Lower - Final v7 (Autodesk Fusion 360 design; units mm, degrees)
Autodesk Fusion 360 part; units mm, degrees
note: some values were not read from the file. Chosen so that the rebuilt part matches the saved one: which bodies a step acts on; which face or edge a step refers to; the sign of a taper.
sketch "Sketch1" plane through (0, 0, 0) normal (0, 1, 0) x (1, 0, 0)
  line L0 (-39.5, 47.5) -> (39.5, 47.5)
  line L1 (49.5, 37.5) -> (49.5, -37.5)
  line L2 (39.5, -47.5) -> (-39.5, -47.5)
  line L3 (-49.5, -37.5) -> (-49.5, 37.5)
  line L4 (-49.5, 47.5) -> (49.5, -47.5) construction
  line L5 (49.5, 47.5) -> (-49.5, -47.5) construction
  arc A0 (-39.5, 47.5) -> (-49.5, 37.5) centre (-39.5, 37.5) ccw
  arc A1 (49.5, 37.5) -> (39.5, 47.5) centre (39.5, 37.5) ccw
  arc A2 (39.5, -47.5) -> (49.5, -37.5) centre (39.5, -37.5) ccw
  arc A3 (-49.5, -37.5) -> (-39.5, -47.5) centre (-39.5, -37.5) ccw
  line L6 (-46.5, -37.5) -> (-46.5, 37.5)
  arc A4 (-39.5, 44.5) -> (-46.5, 37.5) centre (-39.5, 37.5) ccw
  line L7 (-39.5, 44.5) -> (39.5, 44.5)
  arc A5 (46.5, 37.5) -> (39.5, 44.5) centre (39.5, 37.5) ccw
  line L8 (46.5, 37.5) -> (46.5, -37.5)
  arc A6 (39.5, -44.5) -> (46.5, -37.5) centre (39.5, -37.5) ccw
  line L9 (39.5, -44.5) -> (-39.5, -44.5)
  arc A7 (-46.5, -37.5) -> (-39.5, -44.5) centre (-39.5, -37.5) ccw
  line L10 (-44, -37.5) -> (-44, 37.5)
  arc A8 (-39.5, 42) -> (-44, 37.5) centre (-39.5, 37.5) ccw
  line L11 (-39.5, 42) -> (39.5, 42)
  arc A9 (44, 37.5) -> (39.5, 42) centre (39.5, 37.5) ccw
  line L12 (44, 37.5) -> (44, -37.5)
  arc A10 (39.5, -42) -> (44, -37.5) centre (39.5, -37.5) ccw
  line L13 (39.5, -42) -> (-39.5, -42)
  arc A11 (-44, -37.5) -> (-39.5, -42) centre (-39.5, -37.5) ccw
  line L14 (-47, -37.5) -> (-47, 37.5)
  arc A12 (-39.5, 45) -> (-47, 37.5) centre (-39.5, 37.5) ccw
  line L15 (-39.5, 45) -> (39.5, 45)
  arc A13 (47, 37.5) -> (39.5, 45) centre (39.5, 37.5) ccw
  line L16 (47, 37.5) -> (47, -37.5)
  arc A14 (39.5, -45) -> (47, -37.5) centre (39.5, -37.5) ccw
  line L17 (39.5, -45) -> (-39.5, -45)
  arc A15 (-47, -37.5) -> (-39.5, -45) centre (-39.5, -37.5) ccw
  arc A16 (-39.5, 44.4) -> (-46.4, 37.5) centre (-39.5, 37.5) ccw
  line L18 (-46.4, -37.5) -> (-46.4, 37.5)
  arc A17 (-46.4, -37.5) -> (-39.5, -44.4) centre (-39.5, -37.5) ccw
  line L19 (39.5, -44.4) -> (-39.5, -44.4)
  arc A18 (39.5, -44.4) -> (46.4, -37.5) centre (39.5, -37.5) ccw
  line L20 (46.4, 37.5) -> (46.4, -37.5)
  arc A19 (46.4, 37.5) -> (39.5, 44.4) centre (39.5, 37.5) ccw
  line L21 (-39.5, 44.4) -> (39.5, 44.4)
  arc A20 (-39.5, 44.15) -> (-46.15, 37.5) centre (-39.5, 37.5) ccw
  line L22 (-46.15, -37.5) -> (-46.15, 37.5)
  arc A21 (-46.15, -37.5) -> (-39.5, -44.15) centre (-39.5, -37.5) ccw
  line L23 (39.5, -44.15) -> (-39.5, -44.15)
  arc A22 (39.5, -44.15) -> (46.15, -37.5) centre (39.5, -37.5) ccw
  line L24 (46.15, 37.5) -> (46.15, -37.5)
  arc A23 (46.15, 37.5) -> (39.5, 44.15) centre (39.5, 37.5) ccw
  line L25 (-39.5, 44.15) -> (39.5, 44.15)
  arc A24 (-39.5, 45.25) -> (-47.25, 37.5) centre (-39.5, 37.5) ccw
  line L26 (-47.25, -37.5) -> (-47.25, 37.5)
  arc A25 (-47.25, -37.5) -> (-39.5, -45.25) centre (-39.5, -37.5) ccw
  line L27 (39.5, -45.25) -> (-39.5, -45.25)
  arc A26 (39.5, -45.25) -> (47.25, -37.5) centre (39.5, -37.5) ccw
  line L28 (47.25, 37.5) -> (47.25, -37.5)
  arc A27 (47.25, 37.5) -> (39.5, 45.25) centre (39.5, 37.5) ccw
  line L29 (-39.5, 45.25) -> (39.5, 45.25)
  arc A28 (-39.5, 46.5092) -> (-48.5092, 37.5) centre (-39.5, 37.5) ccw
  line L30 (-48.5092, -37.5) -> (-48.5092, 37.5)
  arc A29 (-48.5092, -37.5) -> (-39.5, -46.5092) centre (-39.5, -37.5) ccw
  line L31 (39.5, -46.5092) -> (-39.5, -46.5092)
  arc A30 (39.5, -46.5092) -> (48.5092, -37.5) centre (39.5, -37.5) ccw
  line L32 (48.5092, 37.5) -> (48.5092, -37.5)
  arc A31 (48.5092, 37.5) -> (39.5, 46.5092) centre (39.5, 37.5) ccw
  line L33 (-39.5, 46.5092) -> (39.5, 46.5092)
  arc A32 (-39.5, 44) -> (-46, 37.5) centre (-39.5, 37.5) ccw
  line L34 (-46, -37.5) -> (-46, 37.5)
  arc A33 (-46, -37.5) -> (-39.5, -44) centre (-39.5, -37.5) ccw
  line L35 (39.5, -44) -> (-39.5, -44)
  arc A34 (39.5, -44) -> (46, -37.5) centre (39.5, -37.5) ccw
  line L36 (46, 37.5) -> (46, -37.5)
  arc A35 (46, 37.5) -> (39.5, 44) centre (39.5, 37.5) ccw
  line L37 (-39.5, 44) -> (39.5, 44)
  dimension "d1" = 99
  dimension "d2" = 95
  dimension "d3" = 3
  dimension "d5" = 5.5
  dimension "d7" = 10
  dimension "d31" = 93
  dimension "d32" = -2.5
  dimension "d53" = -3.1
  dimension "d54" = -3.35
  dimension "d57" = -2.25
  dimension "d58" = -0.9908
  dimension "d63" = -3.5
  constraint horizontal L0
  constraint perpendicular L0 L1
  constraint parallel L0 L2
  constraint parallel L1 L3
  constraint coincident L4 origin
  constraint coincident L5 origin
  constraint coincident L4.start L3
  constraint coincident L4.start L0
  constraint tangent L3 A0
  constraint tangent L0 A0
  constraint coincident L5.start L0
  constraint coincident L5.start L1
  constraint tangent L0 A1
  constraint tangent L1 A1
  constraint equal A0 A1
  constraint coincident L4.end L2
  constraint coincident L4.end L1
  constraint tangent L2 A2
  constraint tangent L1 A2
  constraint equal A0 A2
  constraint coincident L5.end L3
  constraint coincident L5.end L2
  constraint tangent L3 A3
  constraint tangent L2 A3
  constraint equal A0 A3
  measures "d1" distance of L4.start L5.start
  measures "d2" distance of L4.start L5.end
  measures "d7" radius of A0
  measures "d31" distance of L6 L8
extrude "Extrude1" add sketch "Sketch1" along normal blind 3 contours L10 A8 L11 A9 L12 A10 L13 A11 | A32 L34 A33 L35 A34 L36 A35 L37 makes body 1
extrude "Extrude2" add sketch "Sketch1" along normal blind 12 from surface at 3 separate body contours L6 A4 L7 A5 L8 A6 L9 A7 | L14 A12 L15 A13 L16 A14 L17 A15 | A16 L18 A17 L19 A18 L20 A19 L21 | A20 L22 A21 L23 A22 L24 A23 L25 | A24 L26 A25 L27 A26 L28 A27 L29 | A28 L30 A29 L31 A30 L32 A31 L33 | A32 L34 A33 L35 A34 L36 A35 L37 makes body 2
extrude "Extrude3" add sketch "Sketch1" along normal blind 15 from surface at 3 contours L6 A4 L7 A5 L8 A6 L9 A7 | L14 A12 L15 A13 L16 A14 L17 A15 | A16 L18 A17 L19 A18 L20 A19 L21 | A20 L22 A21 L23 A22 L24 A23 L25 | A24 L26 A25 L27 A26 L28 A27 L29 | A32 L34 A33 L35 A34 L36 A35 L37 bodies 2 1
ref_plane "WorkPlane1" through (0, 3, 0) normal (0, 1, 0) x (1, 0, 0)
extrude "Extrude4" cut 1 faces at (-13.1667, 3, -14) along direction (0, -1, 0) blind 0.01 on bodies 2 bodies 2
fillet "Fillet1" [suppressed]
draft "Draft1" angle 3 neutral plane through (0, 18, 0) pull (0, 1, 0) 8 faces at (-42.1103, 12.9967, 41.1656) (-44, 12.9967, -12.5) (13.1667, 12.9967, 42) (-42.1103, 12.9967, -41.1656) (13.1667, 7.9933, -42) (42.1103, 12.9967, -41.1656) (44, 12.9967, 12.5) (42.2817, 12.9967, 41.0372) on bodies 2
draft "Draft2" angle -2.1 neutral plane through (0, 3, 0) pull (0, 1, 0) 8 faces at (-41.624, 11, 46.2552) (13.1667, 7, 46.5092) (41.624, 11, 46.2552) (48.5092, 7, -12.5) (48.0137, 11, -40.4466) (-13.1667, 7, -46.5092) (-46.8387, 11, -42.7258) (-48.5092, 7, 12.5) on bodies 2
draft "Draft3" angle 3 neutral plane through (0, 18, 0) pull (0, 1, 0) 8 faces at (-47.2149, 16, 38.2367) (13.1667, 16, 45.25) (45.5919, 16, 42.2907) (47.25, 16, -12.5) (47.2149, 16, -38.2367) (-13.1667, 17, -45.25) (-45.5919, 16, -42.2907) (-47.25, 16, 12.5) on bodies 2
draft "Draft4" angle -3 neutral plane through (0, 0, 0) pull (0, 1, 0) 8 faces at (13.1667, 1, 44) (45.8825, 2, 38.7301) (46, 1, -12.5) (42.4785, 2, -43.2774) (-13.1667, 1, -44) (-41.9158, 2, -43.5344) (-46, 1, 12.5) (-43.2704, 2, 42.7947) on bodies 2
ref_plane "WorkPlane2" through (0, 18, 0) normal (0, 1, 0) x (1, 0, 0)
ref_plane "WorkPlane3" through (0, 36, 0) normal (0, 1, 0) x (0, 0, 1)
fillet "Fillet5" [suppressed]
fillet "Fillet2" [suppressed]
fillet "Fillet3" [suppressed]
sketch "Sketch5" plane through (0, 0, 0) normal (0, 1, 0) x (1, 0, 0)
sketch "Sketch6" plane through (0, 15, 0) normal (0, 1, 0) x (-1, 0, 0)
  line L0 (47.4072, 37.5) -> (47.4072, -37.5)
  arc A0 (39.5, -45.4072) -> (47.4072, -37.5) centre (39.5, -37.5) ccw
  line L1 (39.5, -45.4072) -> (-39.5, -45.4072)
  arc A1 (-47.4072, -37.5) -> (-39.5, -45.4072) centre (-39.5, -37.5) ccw
  line L2 (-47.4072, -37.5) -> (-47.4072, 37.5)
  arc A2 (-39.5, 45.4072) -> (-47.4072, 37.5) centre (-39.5, 37.5) ccw
  line L3 (-39.5, 45.4072) -> (39.5, 45.4072)
  arc A3 (47.4072, 37.5) -> (39.5, 45.4072) centre (39.5, 37.5) ccw
  arc A4 (48.9492, 37.5) -> (39.5, 46.9492) centre (39.5, 37.5) ccw
  line L4 (39.5, 46.9492) -> (-39.5, 46.9492)
  arc A5 (-39.5, 46.9492) -> (-48.9492, 37.5) centre (-39.5, 37.5) ccw
  line L5 (-48.9492, 37.5) -> (-48.9492, -37.5)
  arc A6 (-48.9492, -37.5) -> (-39.5, -46.9492) centre (-39.5, -37.5) ccw
  line L6 (-39.5, -46.9492) -> (39.5, -46.9492)
  arc A7 (39.5, -46.9492) -> (48.9492, -37.5) centre (39.5, -37.5) ccw
  line L7 (48.9492, -37.5) -> (48.9492, 37.5)
  line L8 (-71.5, -69.5) -> (71.5, -69.5)
  line L9 (71.5, -69.5) -> (71.5, 69.5)
  line L10 (71.5, 69.5) -> (-71.5, 69.5)
  line L11 (-71.5, 69.5) -> (-71.5, -69.5)
  line L12 (-71.5, -69.5) -> (71.5, 69.5) construction
  line L13 (71.5, -69.5) -> (-71.5, 69.5) construction
  dimension "d79" = 143
  dimension "d80" = 139
  constraint horizontal L8
  constraint perpendicular L8 L9
  constraint parallel L8 L10
  constraint parallel L9 L11
  constraint coincident L12 origin
  constraint coincident L13 origin
  measures "d79" distance of L9.end L10.end
  measures "d80" distance of L8.end L9.end
extrude "Extrude12" add sketch "Sketch6" along normal blind 25 separate body contours L0 A0 L1 A1 L2 A2 L3 A3 | A4 L4 A5 L5 A6 L6 A7 L7 | L8 L9 L10 L11 makes body 3
sketch "Sketch7" plane through (0, 15, 0) normal (0, -1, 0) x (1, 0, 0)
  line L0 (71.5, -69.5) -> (71.5, 69.5)
  line L1 (71.5, 69.5) -> (-71.5, 69.5)
  line L2 (-71.5, 69.5) -> (-71.5, -69.5)
  line L3 (-71.5, -69.5) -> (71.5, -69.5)
extrude "Extrude13" add 1 faces at (23.8333, 15, -23.1667) along direction (0, -1, 0) blind 25 separate body on bodies 3 makes body 4
combine "Combine3" operation add target body 3 tool bodies 4
combine "Combine4" operation cut target body 3 tool bodies 2 keep tools
ref_plane "WorkPlane5" through (0, 15, 0) normal (0, 1, 0) x (0, 0, 1)
split "Split1" by plane through (0, 15, 0) normal (0, 1, 0) bodies 3 makes body 5 at (23.8333, -10, -23.1667) makes body 6 at (23.8333, 40, -23.1667)
combine "Combine5" operation add target body 6 tool bodies 3
extrude "Extrude14" cut 1 faces at (23.8333, 40, -23.1667) along direction (0, -1, 0) blind 12.01 on bodies 6 bodies 6
copy_body "Body->Comp5" bodies 6 removing the originals makes body 7 in component "Lower-Half"
copy_body "CutPasteBodies1" bodies 5 removing the originals makes body 8 in component "Lower-Half"
copy_body "CutPasteBodies2" bodies 2 removing the originals makes body 9 in component "Lower-Half"
component "Lower-Half" placed x (1, 0, 0) y (0, 1, 0) z (0, 0, 1) at (0, 0, 0)
equation "d22 = 3.0 °"
equation "d23 = 0.0 °"
equation "d24 = 2.1 °"
equation "d25 = 0.0 °"
equation "d26 = 3.0 °"
equation "d27 = 0.0 °"
equation "d28 = 3.0 °"
equation "d29 = 0.0 °"
equation "d79 = 137 mm + 6 mm"
equation "d80 = 133 mm + 6 mm"
equation "d86 = -( 37.01 mm - 25 mm )"
named bodies: "Down", "Up", "Object"
